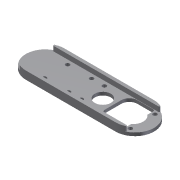
# Autodesk Inventor part: JointC2_
Saved by Autodesk Inventor 2011 SP1 (Build 150282100, 282)
## iProperties
Created: 2012-10-23
Part Number: JointC2_
Document SubType Name: Modeling
Designer: arihon
Density: 1 g/cm^3
Author: arihon
Autodesk Inventor part; units mm, degrees
ref_plane "YZ Plane" through (0, 0, 0) normal (1, 0, 0) x (0, 1, 0)
ref_plane "XZ Plane" through (0, 0, 0) normal (0, 1, 0) x (-1, 0, 0)
ref_plane "XY Plane" through (0, 0, 0) normal (0, 0, 1) x (1, 0, 0)
sketch "スケッチ1" plane through (0, 0, 0) normal (0, 0, 1) x (1, 0, 0)
  line L0 (-40, 12) -> (40, 12)
  line L1 (40, 12) -> (40, -12)
  line L2 (40, -12) -> (-40, -12)
  line L3 (-40, -12) -> (-40, 12)
  point P0 (0, 0)
  dimension "d0" = 80
  dimension "d1" = 24
  dimension "d2" = 12
  dimension "d3" = 40
  constraints: 8 end point, 2 parallel, 1 horizontal, 1 perpendicular
  measures "d0" distance of L1.end L2.end
  measures "d1" distance of L2.end L0.start
  measures "d2" distance from line of L2 point (0, 0)
  measures "d3" distance from line of L3 point (0, 0)
extrude "押し出し1" add sketch "スケッチ1" along normal blind 5
sketch "スケッチ2" plane through (0, 0, 5) normal (0, 0, 1) x (1, 0, 0)
  line L0 (-0.8, 9.8) -> (35, 9.8)
  line L1 (35, 9.8) -> (35, -9.8)
  line L2 (35, -9.8) -> (-0.8, -9.8)
  line L3 (-0.8, -9.8) -> (-0.8, 9.8)
  line L4 (35, 9.8) -> (30.75, 9.8)
  line L5 (30.75, 9.8) -> (30.75, -9.8)
  line L6 (30.75, -9.8) -> (35, -9.8)
  line L7 (35, -9.8) -> (35, 9.8)
  line L8 (30.75, -9.8) -> (14.75, -9.8)
  line L9 (14.75, -9.8) -> (14.75, 9.8)
  line L10 (14.75, 9.8) -> (30.75, 9.8)
  line L11 (30.75, 9.8) -> (30.75, -9.8)
  circle A0 centre (8, 0) radius 5
  line L12 (35, 0) -> (-0.8, 0)
  circle A1 centre (1.8, 7.2) radius 1.25
  circle A2 centre (32.9, 7.7) radius 1.25
  circle A3 centre (1.8, -7.2) radius 1.25
  circle A4 centre (32.9, -7.7) radius 1.25
  line L13 (40, 12) -> (40, -12) projected
  point P0 (0, 0)
  dimension "d6" = 35.8
  dimension "d7" = 19.6
  dimension "d8" = 9.8
  dimension "d10" = 4.25
  dimension "d11" = 16
  dimension "d12" = 10
  dimension "d13" = 27
  dimension "d14" = 14.4
  dimension "d15" = 15.4
  dimension "d16" = 31.1
  dimension "d17" = 2.1
  dimension "d18" = 2.5
  dimension "d19" = 2.5
  dimension "d47" = 5
  constraints: 26 end point, 6 parallel, 5 centre point, 3 horizontal, 3 perpendicular, 2 coincident, 2 midpoint, 2 point on line, 2 symmetric about line, 2 other
  measures "d6" distance of L1.end L2.end
  measures "d7" distance of L2.end L0.start
  measures "d8" distance from line of L2 point (0, 0)
  measures "d10" distance of L6.end L5.end
  measures "d11" distance between parallel lines of L9 L5
  measures "d12" diameter of A0
  measures "d13" distance from line of A0.centre L1
  measures "d14" diameter of point (1.8, 7.2) L12
  measures "d15" diameter of point (32.9, 7.7) L12
  measures "d16" horizontal distance of point (32.9, 7.7) point (1.8, 7.2)
  measures "d17" distance from line of point (32.9, 7.7) L1
  measures "d18" diameter of A1
  measures "d19" diameter of A2
  measures "d47" distance between parallel lines of L13 L7
extrude "押し出し2" cut sketch "スケッチ2" against normal through all contours L0 L5 L12 L9 | L12 L5 L2 L9 | L12 A0 | A0 L12 | A1 | A2 | A3 | A4
fillet "フィレット1" radius 5 2 edges at (14.75, 9.8, 2.5) (14.75, -9.8, 2.5)
fillet "フィレット2" radius 1 2 edges at (30.75, 9.8, 2.5) (30.75, -9.8, 2.5)
sketch "スケッチ5" plane through (0, 0, 5) normal (0, 0, 1) x (1, 0, 0)
  line L0 (40, 12) -> (40, -12) projected
  line L1 (29.75, -9.8) -> (19.75, -9.8) projected
  arc A0 (14.75, -4.8) -> (19.75, -9.8) centre (19.75, -4.8) ccw projected
  line L2 (14.75, -4.8) -> (14.75, 4.8) projected
  arc A1 (19.75, 9.8) -> (14.75, 4.8) centre (19.75, 4.8) ccw projected
  line L3 (19.75, 9.8) -> (29.75, 9.8) projected
  arc A2 (30.75, 8.8) -> (29.75, 9.8) centre (29.75, 8.8) ccw projected
  line L4 (30.75, 8.8) -> (30.75, -8.8) projected
  arc A3 (29.75, -9.8) -> (30.75, -8.8) centre (29.75, -8.8) ccw projected
  circle A4 centre (32.9, -7.7) radius 1.25 projected
  circle A5 centre (1.8, -7.2) radius 1.25 projected
  circle A6 centre (32.9, 7.7) radius 1.25 projected
  circle A7 centre (1.8, 7.2) radius 1.25 projected
  circle A8 centre (8, 0) radius 5 projected
  line L5 (40, 10) -> (-40, 10)
  line L6 (-40, 10) -> (-40, -10)
  line L7 (-40, -10) -> (40, -10)
  line L8 (40, -10) -> (40, 10)
  point P0 (-32.5, 14.4762)
  point P1 (-32.5, -14.4762)
  point P2 (0, 0)
  dimension "d41" = 20
  dimension "d42" = 10
  dimension "d49" = 41.8
  constraints: 8 end point, 2 parallel, 1 horizontal, 1 perpendicular, 1 point on line
  measures "d41" distance between parallel lines of L7 L5
  measures "d42" distance from line of point (0, 0) L5
  measures "d49" distance from line of A7.centre L6
extrude "押し出し4" cut sketch "スケッチ5" against normal blind 3
fillet "フィレット3" radius 12 4 edges at (40, -12, 2.5) (40, 12, 2.5) (-40, -12, 2.5) (-40, 12, 2.5)
fillet "フィレット4" radius 0.5 4 edges at (-34.6333, -10, 3.5) (-34.6333, 10, 3.5) (34.6333, 10, 3.5) (34.6333, -10, 3.5)
sketch "スケッチ6" plane through (0, 0, 2) normal (0, 0, 1) x (1, 0, 0)
  circle A0 centre (32.9, -7.7) radius 1.25 projected
  circle A1 centre (26.72, 0) radius 6.5
  point P0 (0, 0)
  dimension "d52" = 13
  dimension "d53" = 6.18
  constraints: 1 centre point
  measures "d52" diameter of A1
  measures "d53" horizontal distance of A1.centre A0.centre
extrude "押し出し5" cut sketch "スケッチ6" against normal through all contours A1
sketch "スケッチ7" plane through (0, 0, 2) normal (0, 0, 1) x (1, 0, 0)
  circle A0 centre (1.8, -7.2) radius 1.25 projected
  circle A1 centre (1.8, 7.2) radius 1.25 projected
  point P0 (0, 0)
  point P1 (-6.2, 7.2)
  point P2 (-6.2, -7.2)
  point P3 (-21.2, -7.2)
  point P4 (-21.2, 7.2)
  point P5 (-6.2, 7.2)
  point P6 (-21.2, 7.2)
  dimension "d56" = 15
  dimension "d57" = 15
  dimension "d58" = 8
  dimension "d59" = 8
  dimension "d60" = 7.2
  dimension "d61" = 7.2
  dimension "d62" = 7.2
  dimension "d63" = 7.2
  constraints: 2 coincident
  measures "d56" distance of point (-21.2, 7.2) point (-6.2, 7.2)
  measures "d57" distance of point (-21.2, -7.2) point (-6.2, -7.2)
  measures "d58" distance of A1.centre point (-6.2, 7.2)
  measures "d59" distance of A0.centre point (-6.2, -7.2)
  measures "d60" vertical distance of point (0, 0) point (-6.2, 7.2)
  measures "d61" vertical distance of point (0, 0) point (-21.2, 7.2)
  measures "d62" vertical distance of point (-6.2, -7.2) point (0, 0)
  measures "d63" vertical distance of point (-21.2, -7.2) point (0, 0)
hole "Hole2" at (-6.2, 7.2, 2) at (-6.2, -7.2, 2) at (-21.2, -7.2, 2) at (-21.2, 7.2, 2) direction (0, 0, -1) diameter 2.5 end through all
equation "\"d2\" = 0.5 * d1"
equation "\"d3\" = 0.5 * d0"
equation "\"d8\" = 0.5 * d7"
equation "\"d42\" = 0.5 * d41"
equation "\"d57\" = d56"
equation "\"d59\" = d58"
